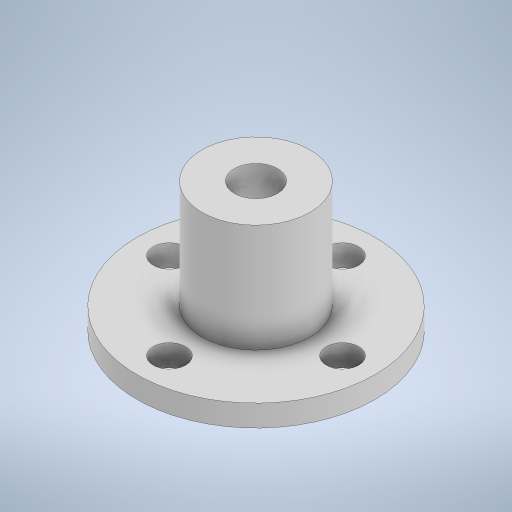
# Autodesk Inventor part: brida
Saved by Autodesk Inventor 2023.1 (Build 271208000, 208)
## iProperties
Created: 2023-05-03
Part Number: brida
Material: Generic
Document SubType Name: Modeling
Designer: felip
Density: 1 g/cm^3
Appearance: Default
Author: felip
Autodesk Inventor part; units mm, degrees
ref_plane "YZ Plane" through (0, 0, 0) normal (1, 0, 0) x (0, 1, 0)
ref_plane "XZ Plane" through (0, 0, 0) normal (0, 1, 0) x (-1, 0, 0)
ref_plane "XY Plane" through (0, 0, 0) normal (0, 0, 1) x (1, 0, 0)
sketch "Sketch1" plane through (0, 0, 0) normal (0, 1, 0) x (-1, 0, 0)
  circle A0 centre (0, 0) radius 11
  circle A1 centre (0, -8) radius 1.5
  circle A2 centre (8, 0) radius 1.5
  circle A3 centre (0, 8) radius 1.5
  circle A4 centre (-8, 0) radius 1.5
  dimension "d0" = 22
  dimension "d15" = 3
  dimension "d18" = 360
  constraints: 5 centre point, 1 coincident, 9 other
  measures "d0" diameter of A0
  measures "d15" diameter of A1
extrude "Extrusion1" add sketch "Sketch1" along normal blind 2
sketch "Sketch2" plane through (0, 2, 0) normal (0, 1, 0) x (1, 0, 0)
  circle A0 centre (0, 0) radius 5
  dimension "d3" = 10
  constraints: 1 centre point, 1 coincident
  measures "d3" diameter of A0
extrude "Extrusion2" add sketch "Sketch2" along normal blind 10
sketch "Sketch3" plane through (0, 12, 0) normal (0, 1, 0) x (1, 0, 0)
  circle A0 centre (0, 0) radius 2
  dimension "d6" = 4
  constraints: 1 centre point, 1 coincident
  measures "d6" diameter of A0
hole "Hole1" at (0, 12, 0) direction (0, -1, 0) diameter 4 end through all
body "Solid1"
